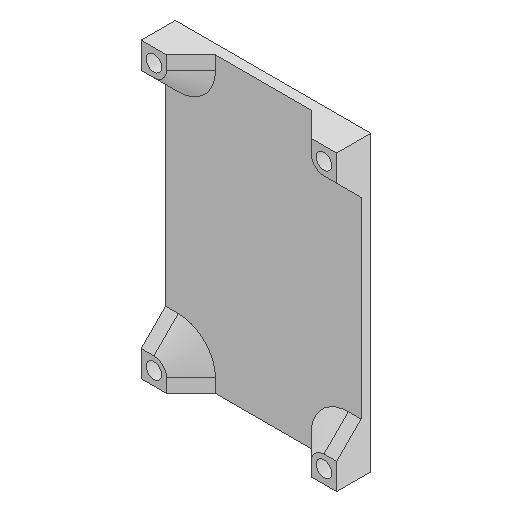
# Autodesk Inventor part: Test_PCB_Board_4x6
Saved by Autodesk Inventor 2026.2 (Build 302298000, 298)
## iProperties
Created: 2026-05-06
Part Number: Test_PCB_Board_4x6
Material: Generic
Document SubType Name: Modeling
Designer: pacoa
Density: 1 g/cm^3
Appearance: Default
Author: pacoa
Autodesk Inventor part; units mm, degrees
ref_plane "YZ Plane" through (0, 0, 0) normal (1, 0, 0) x (0, 1, 0)
ref_plane "XZ Plane" through (0, 0, 0) normal (0, 1, 0) x (-1, 0, 0)
ref_plane "XY Plane" through (0, 0, 0) normal (0, 0, 1) x (1, 0, 0)
sketch "Sketch1" plane through (0, 0, 0) normal (0, 1, 0) x (-1, 0, 0)
  line L0 (0, 0) -> (40, 0)
  line L1 (40, 0) -> (40, -60)
  line L2 (40, -60) -> (0, -60)
  line L3 (0, -60) -> (0, 0)
  circle A0 centre (2.6, -2.75) radius 1.27
  circle A1 centre (37.4, -2.75) radius 1.27
  circle A2 centre (37.4, -57.25) radius 1.27
  circle A3 centre (2.6, -57.25) radius 1.27
  dimension "d1" = 40
  dimension "d2" = 60
  dimension "d15" = 2.54
  dimension "d20" = 2.75
  dimension "d21" = 2.6
  dimension "d22" = 2.54
  dimension "d23" = 2.75
  dimension "d24" = 2.6
  dimension "d25" = 2.54
  dimension "d26" = 2.54
  dimension "d27" = 2.75
  dimension "d28" = 2.75
  dimension "d29" = 2.6
  dimension "d30" = 2.6
  constraints: 8 end point, 4 centre point, 2 parallel, 1 horizontal, 1 perpendicular
  measures "d1" distance of L1.end L2.end
  measures "d2" distance of L0.end L1.end
  measures "d15" diameter of A0
  measures "d20" distance from line of L0 A0.centre
  measures "d21" distance from line of L3 A0.centre
  measures "d22" diameter of A1
  measures "d23" distance from line of L0 A1.centre
  measures "d24" distance from line of L1 A1.centre
  measures "d25" diameter of A2
  measures "d26" diameter of A3
  measures "d27" distance from line of L2 A2.centre
  measures "d28" distance from line of L2 A3.centre
  measures "d29" distance from line of L3 A3.centre
  measures "d30" distance from line of L1 A2.centre
extrude "Extrusion1" add sketch "Sketch1" along normal blind 2 contours L0 L1 L2 L3 | A0 | A1 | A2 | A3
sketch "Sketch2" plane through (0, 0, 0) normal (0, -1, 0) x (1, 0, 0)
  line L0 (-40, 0) -> (0, 0) projected
  line L1 (0, -60) -> (-40, -60) projected
  arc A0 (-5.2, -2.75) -> (-2.6, -5.35) centre (-2.6, -2.75) ccw
  line L2 (0, 0) -> (0, -60) projected
  arc A1 (-2.6, -54.65) -> (-5.2, -57.25) centre (-2.6, -57.25) ccw
  arc A2 (-34.8, -57.25) -> (-37.4, -54.65) centre (-37.4, -57.25) ccw
  line L3 (-40, -60) -> (-40, 0) projected
  arc A3 (-37.4, -5.35) -> (-34.8, -2.75) centre (-37.4, -2.75) ccw
  line L4 (-34.8, -57.25) -> (-34.8, -60)
  line L5 (-34.8, -2.75) -> (-34.8, 0)
  line L6 (-5.2, -57.25) -> (-5.2, -60)
  line L7 (-5.2, -2.75) -> (-5.2, 0)
  line L8 (-37.4, -54.65) -> (-40, -54.65)
  line L9 (0, -5.35) -> (-2.6, -5.35)
  line L10 (-37.4, -5.35) -> (-40, -5.35)
  line L11 (-40, -54.65) -> (-37.4, -54.65)
  line L12 (-2.6, -54.65) -> (0, -54.65)
  constraints: 18 end point, 8 point on circle, 8 point on line, 4 centre point, 4 coincident, 4 tangent, 4 vertical, 3 horizontal
extrude "Extrusion2" add sketch "Sketch2" along normal blind 5 contours L0 L5 A3 L10 L3 | L0 L2 L9 A0 L7 | L8 A2 L4 L1 L3 | L2 L1 L6 A1 L12
sketch "Sketch4" plane through (0, -5, 0) normal (0, -1, 0) x (1, 0, 0)
  arc A0 (-2.6, -54.65) -> (-5.2, -57.25) centre (-2.6, -57.25) ccw projected
  arc A1 (-34.8, -57.25) -> (-37.4, -54.65) centre (-37.4, -57.25) ccw projected
  arc A2 (-5.2, -2.75) -> (-2.6, -5.35) centre (-2.6, -2.75) ccw projected
  arc A3 (-37.4, -5.35) -> (-34.8, -2.75) centre (-37.4, -2.75) ccw projected
  point P0 (0, 0)
  constraints: 4 coincident
hole "Hole2" at (-2.6, -5, -57.25) at (-37.4, -5, -57.25) at (-2.6, -5, -2.75) at (-37.4, -5, -2.75) direction (0, 1, 0) diameter 3.2 depth 4 tip angle 118
chamfer "Chamfer1" distance 5 angle 45 12 edges at (-1.3, 0, -54.65) (-4.4385, 0, -55.4115) (-5.2, 0, -58.625) (-35.5615, 0, -55.4115) (-34.8, 0, -58.625) (-38.7, 0, -54.65) (-35.5615, 0, -4.5885) (-38.7, 0, -5.35) (-34.8, 0, -1.375) (-1.3, 0, -5.35) (-4.4385, 0, -4.5885) (-5.2, 0, -1.375)
equation "\"d23\" = d20"
equation "\"d24\" = d21"
equation "\"d27\" = d23"
equation "\"d28\" = d20"
equation "\"d29\" = d21"
equation "\"d30\" = d21"
body "Solid1"
